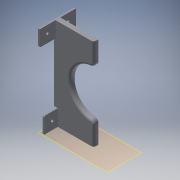
# Autodesk Inventor part: SoporteAmbu
Saved by Autodesk Inventor 2016 (Build 200138000, 138)
## iProperties
Created: 2020-03-19
Part Number: SoporteAmbu
Material: Genérico
Document SubType Name: Modeling
Designer: Andres Gomez
Density: 1 g/cm^3
Appearance: Valor por defecto
Author: Andres Gomez
Autodesk Inventor part; units mm, degrees
ref_plane "YZ Plane" through (0, 0, 0) normal (1, 0, 0) x (0, 1, 0)
ref_plane "XZ Plane" through (0, 0, 0) normal (0, 1, 0) x (-1, 0, 0)
ref_plane "XY Plane" through (0, 0, 0) normal (0, 0, 1) x (1, 0, 0)
ref_plane "Plano de trabajo1" through (0, 0, 0) normal (0, 0, 1) x (1, 0, 0)
sketch "Boceto1" plane through (0, 0, 0) normal (0, 0, 1) x (1, 0, 0)
  line L0 (-72.9949, 0) -> (-72.9949, 3)
  line L1 (-72.9949, 3) -> (-72.9949, -3)
  line L2 (-72.9949, -3) -> (-22.9949, -3)
  line L3 (-22.9949, -3) -> (-22.9949, 3)
  line L4 (-22.9949, 3) -> (-72.9949, 3)
  point P0 (0, 0)
  dimension "d0" = 3
  dimension "d1" = 6
  dimension "d2" = 50
  dimension "d3" = 90
  dimension "d4" = 6
  constraints: 10 end point, 2 perpendicular, 1 point on line, 1 vertical
  measures "d0" distance of L0.start L0.end
  measures "d1" distance of L0.end L1.end
  measures "d2" distance of L1.end L2.end
  measures "d3" angle of L2 L1
  measures "d4" distance of L2.end L3.end
extrude "Extrusión1" add sketch "Boceto1" along normal blind 115
sketch "Boceto2" plane through (-72.9949, 3, 0) normal (0, 1, 0) x (1, 0, 0)
  line L0 (0, 0) -> (0, -115) projected
  line L1 (0, 0) -> (3, 0)
  line L2 (3, 0) -> (3, -20.4)
  line L3 (3, -20.4) -> (0, -20.4)
  line L4 (0, -20.4) -> (0, 0)
  point P0 (72.9949, 0)
  dimension "d7" = 3
  dimension "d8" = 20.4
  constraints: 8 end point, 2 parallel, 1 horizontal, 1 perpendicular
  measures "d7" distance of L2.end L3.end
  measures "d8" distance of L1.end L2.end
extrude "Extrusión2" cut sketch "Boceto2" against normal blind 6
sketch "Boceto3" plane through (-72.9949, 3, 115) normal (0, 1, 0) x (1, 0, 0)
  line L0 (3, 115) -> (50, 115) projected
  line L1 (3, 115) -> (5, 115)
  line L2 (5, 115) -> (5, 94.6)
  line L3 (5, 94.6) -> (3, 94.6)
  line L4 (3, 94.6) -> (3, 115)
  point P0 (72.9949, 115)
  dimension "d11" = 2
  dimension "d12" = 20.4
  constraints: 8 end point, 2 parallel, 1 horizontal, 1 perpendicular
  measures "d11" distance of L2.end L3.end
  measures "d12" distance of L1.end L2.end
extrude "Extrusión3" add sketch "Boceto3" along normal blind 17
sketch "Boceto5" plane through (-72.9949, -3, 115) normal (0, -1, 0) x (1, 0, 0)
  line L0 (3, -94.6) -> (0, -94.6) projected
  line L1 (3, -94.6) -> (5, -94.6)
  line L2 (5, -94.6) -> (5, -115)
  line L3 (5, -115) -> (3, -115)
  line L4 (3, -115) -> (3, -94.6)
  point P0 (72.9949, -115)
  dimension "d15" = 2
  dimension "d16" = 20.4
  constraints: 8 end point, 2 parallel, 1 horizontal, 1 perpendicular
  measures "d15" distance of L2.end L3.end
  measures "d16" distance of L1.end L2.end
extrude "Extrusión4" add sketch "Boceto5" along normal blind 17
fillet "Empalme1" radius 2 2 edges at (-68.9949, -20, 20.4) (-68.9949, 20, 20.4)
sketch "Boceto6" plane through (-69.9949, -20, 0) normal (-1, 0, 0) x (0, 0, 1)
  circle A0 centre (10.1353, 9.969) radius 1.7
  circle A1 centre (10.1353, 30.0745) radius 1.7
  point P0 (0, 20)
  dimension "d20" = 3.4
  dimension "d21" = 3.4
  constraints: 2 centre point
  measures "d20" diameter of A0
  measures "d21" diameter of A1
extrude "Extrusión5" cut sketch "Boceto6" against normal blind 2
sketch "Boceto7" plane through (-72.9949, -3, 115) normal (0, -1, 0) x (1, 0, 0)
  line L0 (0, 0) -> (2, 0)
  line L1 (2, 0) -> (2, -20)
  line L2 (2, -20) -> (0, -20)
  line L3 (0, -20) -> (0, 0)
  point P0 (72.9949, -115)
  dimension "d24" = 2
  dimension "d25" = 20
  constraints: 8 end point, 2 parallel, 1 horizontal, 1 perpendicular
  measures "d24" distance of L1.end L2.end
  measures "d25" distance of L0.end L1.end
extrude "Extrusión6" add sketch "Boceto7" along normal blind 20
sketch "Boceto8" plane through (-72.9949, 3, 115) normal (0, 1, 0) x (1, 0, 0)
  line L0 (2, 20) -> (2, 0) projected
  line L1 (0, 0) -> (2, 0)
  line L2 (2, 0) -> (2, 20)
  line L3 (2, 20) -> (0, 20)
  line L4 (0, 20) -> (0, 0)
  point P0 (72.9949, 115)
  dimension "d28" = 2
  dimension "d29" = 20
  constraints: 8 end point, 2 parallel, 1 horizontal, 1 perpendicular
  measures "d28" distance of L3.end L0.start
  measures "d29" distance of L0.start L1.end
extrude "Extrusión7" add sketch "Boceto8" along normal blind 20
sketch "Boceto9" plane through (-72.9949, -3, 20.4) normal (-1, 0, 0) x (0, 0, 1)
  circle A0 centre (85.3122, 16) radius 1.7
  circle A1 centre (85.3122, -10.078) radius 1.7
  point P0 (-20.4, 3)
  dimension "d32" = 3.4
  dimension "d33" = 3.4
  constraints: 2 centre point
  measures "d32" diameter of A0
  measures "d33" diameter of A1
extrude "Extrusión8" cut sketch "Boceto9" against normal blind 20
fillet "Empalme2" radius 2 2 edges at (-71.9949, 23, 95) (-71.9949, -23, 95)
sketch "Boceto10" plane through (-22.9949, 3, 115) normal (0, 1, 0) x (1, 0, 0)
  line L0 (0, 115) -> (0, 0) projected
  line L1 (0, 115) -> (0, 57.5)
  line L2 (0, 57.5) -> (0, 86.25)
  line L3 (0, 57.5) -> (28.75, 57.5) construction
  line L4 (0, 86.25) -> (0, 28.75)
  line L5 (-50, 94.6) -> (-50, 20) projected
  line L6 (-50, 57.3) -> (-30, 57.3)
  line L7 (-50, 57.3) -> (-30, 57.3) construction
  line L8 (0, 86.25) -> (0, 28.75)
  arc A0 (0, 86.25) -> (0, 28.75) centre (-1.2246, 57.5) ccw
  point P0 (22.9949, 115)
  dimension "d37" = 57.5
  dimension "d39" = 28.75
  dimension "d40" = 90
  dimension "d41" = 57.5
  dimension "d42" = 0
  dimension "d43" = 20
  dimension "d44" = 0
  constraints: 14 end point, 3 horizontal, 3 point on circle, 2 collinear, 2 equal length, 2 midpoint, 1 centre point, 1 vertical
  measures "d37" distance of L0.start L1.end
  measures "d39" distance of L1.end L2.end
  measures "d40" angle of L3 L2
  measures "d41" distance of L2.end L4.end
  measures "d42" distance between parallel lines of L4 L2
  measures "d43" distance of L6.start L6.end
  measures "d44" distance between parallel lines of L6 L7
extrude "Extrusión9" cut sketch "Boceto10" against normal blind 20
fillet "Empalme3" radius 5 2 edges at (-22.9949, 0, 86.25) (-22.9949, 0, 28.75)
fillet "Empalme4" radius 3 5 edges at (-22.9949, -3, 11.9678) (-24.267, -3, 87.7323) (-24.267, -3, 27.2677) (-52.9955, -3, 57.5) (-22.9949, -3, 103.0322)
